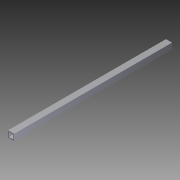
# Autodesk Inventor part: 26 tubing
Saved by Autodesk Inventor 2011 (Build 150239000, 239)
## iProperties
Created: 2013-01-17
Part Number: 26 tubing
Document SubType Name: Modeling
Designer: RESHIRAM
Density: 1 g/cm^3
Author: RESHIRAM
Autodesk Inventor part; units mm, degrees
ref_plane "YZ Plane" through (0, 0, 0) normal (1, 0, 0) x (0, 1, 0)
ref_plane "XZ Plane" through (0, 0, 0) normal (0, 1, 0) x (-1, 0, 0)
ref_plane "XY Plane" through (0, 0, 0) normal (0, 0, 1) x (1, 0, 0)
sketch "Sketch1" plane through (0, 0, 0) normal (0, 0, 1) x (1, 0, 0)
  line L0 (-25.4, 0) -> (0, 0)
  line L1 (0, 0) -> (0, 25.4)
  line L2 (0, 25.4) -> (-25.4, 25.4)
  line L3 (-25.4, 25.4) -> (-25.4, 0)
  line L4 (-22.225, 3.175) -> (-3.175, 3.175)
  line L5 (-3.175, 3.175) -> (-3.175, 22.225)
  line L6 (-3.175, 22.225) -> (-22.225, 22.225)
  line L7 (-22.225, 22.225) -> (-22.225, 3.175)
  dimension "d0" = 25.4
  dimension "d1" = 25.4
  dimension "d2" = 19.05
  dimension "d3" = 19.05
  constraints: 16 end point, 4 parallel, 2 horizontal, 2 perpendicular
  measures "d0" distance of L2.end L1.end
  measures "d1" distance of L1.end L0.end
  measures "d2" distance of L6.end L5.end
  measures "d3" distance of L5.end L4.end
extrude "Extrusion1" add sketch "Sketch1" along normal mid plane 660.4
body "Solid1"
